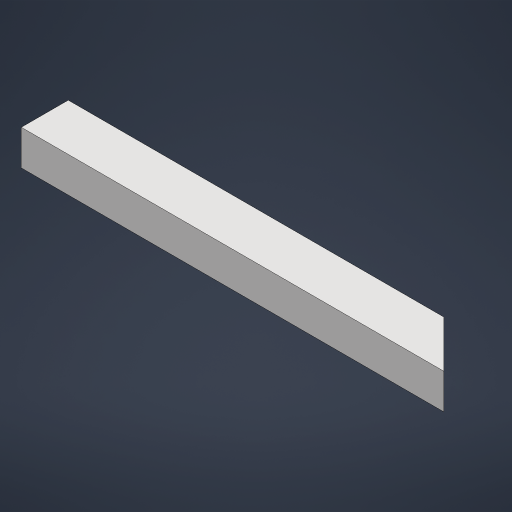
# Autodesk Inventor part: RiserM
Saved by Autodesk Inventor 2023.2 (Build 272271000, 271)
## iProperties
Created: 2022-11-23
Part Number: RiserM
Material: Generic
Document SubType Name: Modeling
Designer: awelt
Mass: 835.74 g
Surface Area: 814.467 cm^2
Volume: 835.74 cm^3
Density: 1 g/cm^3
Appearance: Default
RuleStatus: InUse
BeforeDocSave0: file://C:\Users\awelt\Documents\Inventor\iLogic_Rules\BoundingStore
DocClose0: file://C:\Users\awelt\Documents\Inventor\iLogic_Rules\BoundingStore
Author: awelt
BoundingBL1: 1 1/2
BoundingBL2: 2
BoundingBL3: 18
BoundingCF: 0.031
Autodesk Inventor part; units mm, degrees
ref_plane "YZ Plane" through (0, 0, 0) normal (1, 0, 0) x (0, 1, 0)
ref_plane "XZ Plane" through (0, 0, 0) normal (0, 1, 0) x (-1, 0, 0)
ref_plane "XY Plane" through (0, 0, 0) normal (0, 0, 1) x (1, 0, 0)
sketch "Sketch2" plane through (0, 0, 0) normal (0, 1, 0) x (-1, 0, 0)
  line L0 (0, 0) -> (-457.2, 0)
  line L1 (-457.2, 0) -> (-457.2, -50.8)
  line L2 (-457.2, -50.8) -> (0, -50.8)
  line L3 (0, -50.8) -> (0, 0)
  line L4 (-457.2, 0) -> (-406.4, -50.8)
  line L5 (-457.2, 0) -> (-385.358, 0) construction
  dimension "d3" = 457.2
  dimension "d4" = 50.8
  dimension "d5" = 45
  constraints: 12 end point, 2 horizontal, 2 parallel, 1 equal length, 1 perpendicular, 1 point on line
  measures "d3" distance of L2.end L1.end
  measures "d4" distance of L1.end L0.end
  measures "d5" angle of L4 L5
extrude "Extrusion1" add sketch "Sketch2" along normal blind 38.1 contours L3 L2 L4 L0
body "Solid1"
